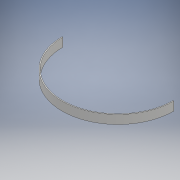
# Autodesk Inventor part: 鋁底板-半圓
Saved by Autodesk Inventor 2018 (Build 220112000, 112)
## iProperties
Created: 2026-01-20
Part Number: 鋁底板-半圓
Material: 一般
Document SubType Name: Modeling
Designer: User
Density: 1 g/cm^3
Appearance: 預設
Author: User
Autodesk Inventor part; units mm, degrees
ref_plane "YZ Plane" through (0, 0, 0) normal (1, 0, 0) x (0, 1, 0)
ref_plane "XZ Plane" through (0, 0, 0) normal (0, 1, 0) x (-1, 0, 0)
ref_plane "XY Plane" through (0, 0, 0) normal (0, 0, 1) x (1, 0, 0)
sketch "草圖1" plane through (0, 0, 0) normal (0, 0, 1) x (1, 0, 0)
  circle A0 centre (0, 0) radius 317
  circle A1 centre (0, 0) radius 322
  dimension "d0" = 634
  dimension "d1" = 644
  constraints: 2 centre point, 2 coincident
  measures "d0" diameter of A0
  measures "d1" diameter of A1
extrude "擠出1" add sketch "草圖1" along normal blind 50
sketch "草圖2" plane through (0, 0, 50) normal (0, 0, 1) x (1, 0, 0)
  line L0 (-488.5314, 349.6941) -> (538.4038, 349.6941)
  line L1 (538.4038, 349.6941) -> (538.4038, 0)
  line L2 (538.4038, 0) -> (-488.5314, 0)
  line L3 (-488.5314, 0) -> (-488.5314, 349.6941)
  point P0 (0, 0)
  dimension "d4" = 0
  constraints: 8 end point, 2 parallel, 1 horizontal, 1 perpendicular
  measures "d4" distance from line of point (0, 0) L2
extrude "擠出2" cut sketch "草圖2" against normal blind 50
